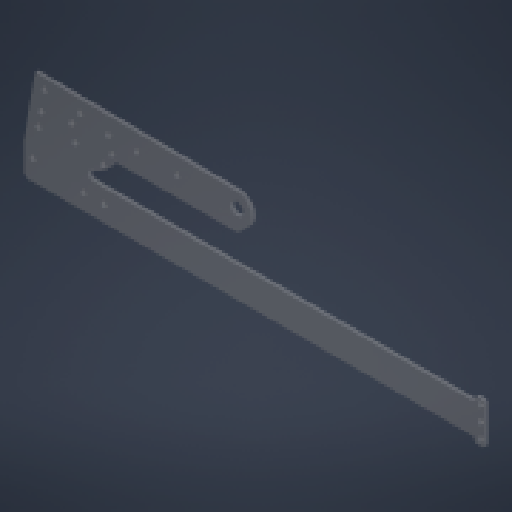
# Autodesk Inventor part: RACK_GUIDES
Saved by Autodesk Inventor 2026.2 (Build 302298010, 298A)
## iProperties
Created: 2026-04-01
Part Number: RACK_GUIDES
Material: Polycarbonate, PC 1000, Clear
Document SubType Name: Sheet Metal
Designer: 4aida
Density: 1.20131 g/cm^3
Sheet Metal Rule: Default
Appearance: Lexan (Clear)
Author: 4aida
Autodesk Inventor part; units mm, degrees
ref_plane "YZ Plane" through (0, 0, 0) normal (1, 0, 0) x (0, 1, 0)
ref_plane "XZ Plane" through (0, 0, 0) normal (0, 1, 0) x (-1, 0, 0)
ref_plane "XY Plane" through (0, 0, 0) normal (0, 0, 1) x (1, 0, 0)
sketch "Sketch1" plane through (0, 0, 0) normal (0, 0, 1) x (1, 0, 0)
  line L0 (279.4704, -19.05) -> (-282.4704, -19.05)
  line L1 (-282.4704, -19.05) -> (-282.4704, 19.05)
  line L2 (-282.4704, 19.05) -> (279.4704, 19.05)
  line L3 (282.4704, -19.05) -> (-282.4704, 19.05) construction
  line L4 (-282.4704, -19.05) -> (282.4704, 19.05) construction
  line L5 (292.1704, -25.05) -> (285.4704, -25.05)
  line L6 (285.4704, 25.05) -> (292.1704, 25.05)
  line L7 (295.1704, 22.05) -> (295.1704, -22.05)
  line L8 (295.1704, -25.05) -> (282.4704, 25.05) construction
  line L9 (282.4704, -25.05) -> (295.1704, 25.05) construction
  line L10 (282.4704, -22.05) -> (282.4704, -22.05)
  line L11 (282.4704, 22.05) -> (282.4704, 22.05)
  arc A0 (279.4704, 19.05) -> (282.4704, 22.05) centre (279.4704, 22.05) ccw
  arc A1 (285.4704, 25.05) -> (282.4704, 22.05) centre (285.4704, 22.05) ccw
  arc A2 (295.1704, 22.05) -> (292.1704, 25.05) centre (292.1704, 22.05) ccw
  arc A3 (292.1704, -25.05) -> (295.1704, -22.05) centre (292.1704, -22.05) ccw
  arc A4 (282.4704, -22.05) -> (285.4704, -25.05) centre (285.4704, -22.05) ccw
  arc A5 (282.4704, -22.05) -> (279.4704, -19.05) centre (279.4704, -22.05) ccw
  point P0 (0, 0)
  point P1 (288.8204, 0)
  point P2 (282.4704, 0)
  point P3 (295.1704, 0)
  dimension "d0" = 12.7
  dimension "d1" = 577.6407
  dimension "d2" = 6
  dimension "d3" = 38.1
  dimension "d4" = 3
  measures "d0" distance of L8.end L9.end
  measures "d1" distance between parallel lines of L7 L1
  measures "d2" distance between parallel lines of L2 L6
  measures "d3" distance between parallel lines of L2 L0
  measures "d4" radius of A0
extrude "Plate1" add sketch "Sketch1" along normal blind 4.7625
sketch "Sketch2" plane through (0, 0, 0) normal (0, 0, -1) x (-1, 0, 0)
  line L0 (-288.8204, -19.05) -> (-288.8204, 19.05)
  line L1 (-295.1704, -22.05) -> (-295.1704, 22.05) projected
  line L2 (-288.8204, 0) -> (-295.1704, 0)
  point P0 (0, 0)
  dimension "d6" = 6.35
  dimension "d7" = 38.1
  constraints: 4 end point, 2 midpoint, 1 coincident, 1 parallel, 1 perpendicular
  measures "d6" distance between parallel lines of L1 L0
  measures "d7" distance of L0.start L0.end
hole "Hole1" at (288.8204, -19.05, 0) at (288.8204, 0, 0) at (288.8204, 19.05, 0) direction (0, 0, 1) diameter 5.1054 depth 4.7625 tip angle 118 clearance for "Flat Head Machine Screw (82)" size "#10" standard "Ansi Unified Screw Threads"
sketch "Sketch3" plane through (0, 0, 0) normal (0, 0, -1) x (-1, 0, 0)
  line L0 (268.0066, 101.0778) -> (282.4704, 19.05)
  line L1 (180.2314, 85.6006) -> (268.0066, 101.0778)
  arc A0 (180.2314, 85.6006) -> (176.9524, 83.8547) centre (181.2732, 79.6918) ccw
  arc A1 (176.9524, 83.8547) -> (183.5568, 37.0593) centre (198.5568, 63.04) ccw
  line L2 (-279.4704, 19.05) -> (282.4704, 19.05)
  line L3 (282.4704, 19.05) -> (214.7497, 19.05)
  line L4 (282.4704, 19.05) -> (282.4704, -19.05)
  arc A2 (196.0756, 19.05) -> (196.0756, 31.05) centre (196.0756, 25.05) ccw
  line L5 (196.0756, 31.05) -> (193.9651, 31.05)
  line L6 (193.9651, 31.05) -> (183.5568, 37.0593)
  arc A3 (169.2665, 76.5071) -> (165.9875, 74.7612) centre (170.3084, 70.5983) ccw
  line L7 (169.8961, 54.1762) -> (13.9062, 54.1762)
  arc A4 (15.2621, 98.6253) -> (1.9766, 66.1058) centre (15.447, 79.5762) ccw
  line L8 (268.0066, 101.0778) -> (15.2621, 98.6253)
  line L9 (13.9062, 54.1762) -> (1.9766, 66.1058)
  circle A5 centre (15.447, 79.5762) radius 7.9502
  line L10 (282.4704, 19.05) -> (-279.4704, 19.05)
  point P0 (0, 0)
  point P1 (187.5919, 53.9466)
  dimension "d16" = 43.99
  dimension "d17" = 80
  dimension "d18" = 83.9136
  dimension "d19" = 30
  dimension "d20" = 6
  dimension "d21" = 83.2932
  dimension "d28" = 12
  dimension "d29" = 86.3948
  dimension "d30" = 30
  dimension "d44" = 6
  dimension "d45" = 25.4
  dimension "d46" = 38.1
  dimension "d47" = 135
  dimension "d48" = 15.9004
  dimension "d49" = 35.1262
  dimension "d50" = 252.4564
  measures "d16" distance from line of L2 A1.centre
  measures "d17" angle of L2 L0
  measures "d18" distance from line of L4 A1.centre
  measures "d19" radius of A1
  measures "d20" radius of A0
  measures "d21" distance from line of L0.end L1
  measures "d28" diameter of A2
  measures "d29" distance from line of L4 A2.centre
  measures "d30" angle of L2 L6
  measures "d44" radius of A3
  measures "d45" distance from line of L7 A4.centre
  measures "d46" diameter of A4
  measures "d47" angle of L7 L9
  measures "d48" diameter of A5
  measures "d49" distance between parallel lines of L7 L2
  measures "d50" distance from line of L0 A5.centre
sheet face with bend "Face2" sketch "Sketch3" thickness 4.7625 toward (0, 0, 1) bend radius 4.7625
bend "Bend1"
fillet "Corner Round1" radius 6.35 5 edges at (-282.4704, 19.05, 2.3813) (-282.4704, -19.05, 2.3813) (-193.9651, 31.05, 2.3813) (-13.9062, 54.1762, 2.3813) (-169.8961, 54.1762, 2.3813)
sketch "Sketch4" plane through (0, 0, 0) normal (0, 0, -1) x (-1, 0, 0)
  line L0 (282.3739, 19.5971) -> (268.0066, 101.0778) projected
  arc A0 (169.8961, 54.1762) -> (183.5568, 37.0593) centre (198.5568, 63.04) ccw projected
  circle A1 centre (198.5568, 63.04) radius 25.4
  line L1 (177.7503, 77.6089) -> (213.1256, 83.8465)
  line L2 (213.1256, 83.8465) -> (183.9879, 42.2336)
  line L3 (183.9879, 42.2336) -> (219.3632, 48.4712)
  line L4 (173.5426, 58.6294) -> (223.5709, 67.4507)
  line L5 (282.3739, 19.5971) -> (268.0066, 101.0778) projected
  line L6 (262.1156, 61.3512) -> (265.4236, 42.5907)
  line L7 (196.0756, 19.05) -> (-279.4704, 19.05) projected
  line L8 (268.0066, 101.0778) -> (15.2621, 98.6253) projected
  line L9 (16.5365, 54.1762) -> (165.5437, 54.1762) projected
  circle A2 centre (15.447, 79.5762) radius 7.9502 projected
  point P0 (0, 0)
  point P1 (257.7049, 86.3654)
  point P2 (272.0396, 5.0695)
  point P3 (208.4539, 0)
  point P4 (182.662, 0)
  point P5 (142.447, 77.1409)
  point P6 (91.647, 77.1409)
  dimension "d31" = 25.4
  dimension "d33" = 12.7
  dimension "d34" = 12.7
  dimension "d42" = 50.8
  dimension "d43" = 45
  dimension "d51" = 5.2605
  dimension "d52" = 19.05
  dimension "d53" = 38.1
  dimension "d54" = 19.05
  dimension "d55" = 19.05
  dimension "d56" = 76.2
  dimension "d57" = 101.6
  dimension "d58" = 22.2246
  dimension "d60" = 44.4491
  dimension "d61" = 50.8
  dimension "d62" = 76.2
  constraints: 10 end point, 9 coincident, 6 point on circle, 2 midpoint, 2 parallel, 2 point on line, 1 centre point, 1 horizontal alignment, 1 perpendicular
  measures "d31" distance of L6.start point (257.705, 86.365)
  measures "d33" distance from line of L0 point (257.705, 86.365)
  measures "d34" distance from line of L0 L6.start
  measures "d42" diameter of A1
  measures "d43" angle of L1 L2
  measures "d51" distance from line of L1 point (257.705, 86.365)
  measures "d52" distance of L6.start L6.end
  measures "d53" distance of point (272.04, 5.069) point (265.424, 42.591)
  measures "d54" distance from line of L7 point (182.662, 0)
  measures "d55" distance from line of point (208.454, 0) L7
  measures "d56" distance from line of point (208.454, 0) L0
  measures "d57" distance from line of L0 point (182.662, 0)
  measures "d58" distance from line of L8 point (91.647, 77.141)
  measures "d60" distance from line of L9 L8.end
  measures "d61" distance of point (142.447, 77.141) point (91.647, 77.141)
  measures "d62" horizontal distance of A2.centre point (91.647, 77.141)
hole "Hole2" at (-257.7049, 86.3654, 0) at (-262.1156, 61.3512, 0) at (-177.7503, 77.6089, 0) at (-173.5426, 58.6294, 0) at (-183.9879, 42.2336, 0) at (-219.3632, 48.4712, 0) at (-223.5709, 67.4507, 0) at (-213.1256, 83.8465, 0) at (-272.0396, 5.0695, 0) at (-265.4236, 42.5907, 0) at (-208.4539, 0, 0) at (-182.662, 0, 0) at (-142.447, 77.1409, 0) at (-91.647, 77.1409, 0) direction (0, 0, 1) diameter 5.105 end through all clearance for "Flat Head Machine Screw (82)" size "#10" standard "Ansi Unified Screw Threads"
equation "\"d13\" = Thickness"
equation "\"d33\" = d32"
equation "\"d34\" = d32"
equation "\"d58\" = 0.5 * d60"
equation "\"d40\" = Thickness"
equation "\"d5\" = Thickness"
equation "\"d22\" = BendRadius"
equation "\"d23\" = BendReliefWidth"
equation "\"d25\" = MinimumRemnant"
equation "\"d24\" = BendReliefDepth"
equation "\"d26\" = TransitionRadius"
equation "\"BendRadius\" = Thickness"
equation "\"BendReliefWidth\" = Thickness"
equation "\"BendReliefDepth\" = 0.5 * Thickness"
equation "\"CornerReliefSize\" = 4 * Thickness"
equation "\"MinimumRemnant\" = 2 * Thickness"
equation "\"TransitionRadius\" = BendRadius"
equation "\"JacobiRadiusSize\" = BendRadius"
equation "\"GapSize\" = Thickness"
equation "\"Thickness\" = 4.7625"
equation "\"d32\" = 12.7"
body "Solid1"
